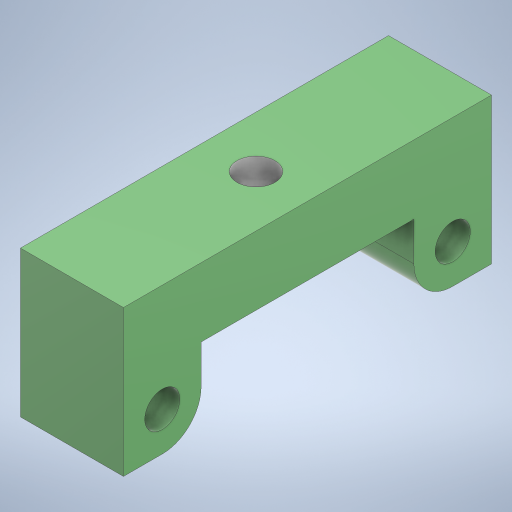
# Autodesk Inventor part: sostenedor_part2
Saved by Autodesk Inventor 2023.2 (Build 272271030, 271C)
## iProperties
Created: 2023-03-04
Part Number: sostenedor_part2
Material: Generic
Document SubType Name: Modeling
Designer: Cris Pat
Density: 1 g/cm^3
Appearance: Default
Author: Cris Pat
Autodesk Inventor part; units mm, degrees
ref_plane "YZ Plane" through (0, 0, 0) normal (1, 0, 0) x (0, 1, 0)
ref_plane "XY Plane" through (0, 0, 0) normal (0, 0, 1) x (1, 0, 0)
sketch "Sketch3" plane through (0, 0, 0) normal (1, 0, 0) x (0, 1, 0)
  circle A0 centre (0, 0) radius 5.65 construction
  line L0 (-5.65, 0) -> (-5.65, 5.65)
  line L1 (0, -5.65) -> (5.65, -5.65)
  arc A1 (-5.65, 0) -> (0, -5.65) centre (0, 0) ccw
  line L2 (-5.65, 5.65) -> (5.65, 5.65)
  line L3 (5.65, -21.15) -> (-5.65, -21.15) construction
  line L4 (5.65, 5.65) -> (15.65, 5.65)
  line L5 (15.65, 5.65) -> (15.65, -21.15)
  line L6 (5.65, -5.65) -> (5.65, -21.15)
  line L7 (15.65, -21.15) -> (5.65, -21.15) construction
  circle A2 centre (0, 0) radius 2.55
  line L8 (-5.65, -42.3) -> (-5.65, -47.95)
  arc A3 (0, -36.65) -> (-5.65, -42.3) centre (0, -42.3) ccw
  line L9 (0, -36.65) -> (5.65, -36.65)
  line L10 (-5.65, -47.95) -> (5.65, -47.95)
  line L11 (5.65, -47.95) -> (15.65, -47.95)
  line L12 (15.65, -47.95) -> (15.65, -21.15)
  line L13 (5.65, -36.65) -> (5.65, -21.15)
  circle A4 centre (0, -42.3) radius 2.55
  dimension "d19" = 11.3
  dimension "d20" = 5.65
  dimension "d22" = 21.15
  dimension "d23" = 10
  dimension "d24" = 10
  dimension "d25" = 11.3
  dimension "d26" = 5.1
  constraints: 28 end point, 8 symmetric about line, 6 point on circle, 5 centre point, 5 horizontal, 3 coincident, 3 tangent, 2 vertical alignment, 1 concentric, 1 perpendicular, 1 point on line, 1 vertical, 2 other
  measures "d19" distance of L2.end L1.end
  measures "d20" radius of A1
  measures "d22" distance from line of A1.centre L3
  measures "d23" distance of L2.end L4.end
  measures "d24" distance between parallel lines of L6 L5
  measures "d25" distance between parallel lines of L0 L6
  measures "d26" diameter of A2
extrude "Extrusion2" add sketch "Sketch3" along normal mid plane 15
ref_plane "Work Plane1" through (0, 5.5, 0) normal (0, 1, 0) x (-1, 0, 0)
sketch "Sketch4" plane through (0, 5.5, 0) normal (0, 1, 0) x (-1, 0, 0)
  line L0 (7.5, -36.65) -> (-7.5, -36.65) construction
  line L1 (-7.5, -5.65) -> (-7.5, -36.65) construction
  line L2 (-7.5, -5.65) -> (7.5, -5.65) construction
  line L3 (7.5, -36.65) -> (7.5, -5.65) construction
  line L4 (7.5, -36.65) -> (-7.5, -36.65) construction
  line L5 (0, -36.65) -> (0, -5.65) construction
  line L6 (-7.5, -5.65) -> (-7.5, -36.65) construction
  line L7 (-7.5, -21.15) -> (7.5, -21.15) construction
  circle A0 centre (0, -21.15) radius 2.75
  circle A1 centre (0, -21.15) radius 4.05
  point P0 (0, 0)
  dimension "d30" = 5.5
  dimension "d31" = 8.1
  constraints: 5 midpoint, 4 end point, 2 centre point, 1 coincident
  measures "d30" diameter of A0
  measures "d31" diameter of A1
extrude "Extrusion3" cut sketch "Sketch4" along normal through all both and the other way through all contours A0
extrude "Extrusion4" cut sketch "Sketch4" along normal mid plane 3.1
body "Solid2"
